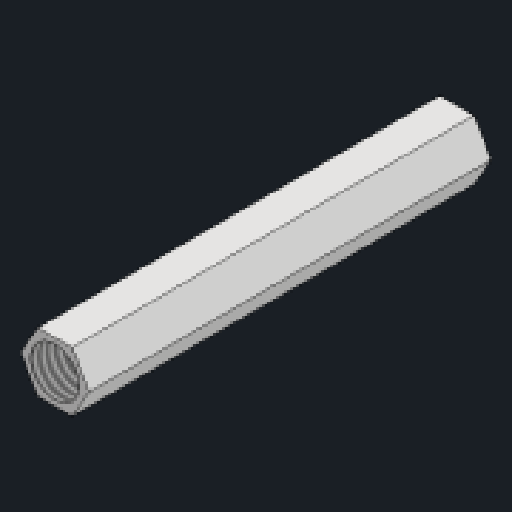
# Autodesk Inventor part: M3 x 25mm Threaded Spacer
Saved by Autodesk Inventor 2023.2 (Build 272271030, 271C)
## iProperties
Created: 2024-02-28
Part Number: M3 x 25mm Threaded Spacer
Material: Brass, Soft Yellow
Document SubType Name: Modeling
Designer: robpl
Density: 8.47 g/cm^3
Appearance: Brass - Satin
Author: robpl
Autodesk Inventor part; units mm, degrees
ref_plane "YZ Plane" through (0, 0, 0) normal (1, 0, 0) x (0, 1, 0)
ref_plane "XZ Plane" through (0, 0, 0) normal (0, 1, 0) x (-1, 0, 0)
ref_plane "XY Plane" through (0, 0, 0) normal (0, 0, 1) x (1, 0, 0)
sketch "Sketch1" plane through (0, 0, 0) normal (0, 0, 1) x (1, 0, 0)
  line L0 (-1.0681, -1.85) -> (-2.1362, 0)
  line L1 (-2.1362, 0) -> (-1.0681, 1.85)
  line L2 (-1.0681, 1.85) -> (1.0681, 1.85)
  line L3 (1.0681, 1.85) -> (2.1362, 0)
  line L4 (2.1362, 0) -> (1.0681, -1.85)
  line L5 (1.0681, -1.85) -> (-1.0681, -1.85)
  circle A0 centre (0, 0) radius 1.5
  dimension "d0" = 3.7
  dimension "d3" = 3
  constraints: 12 end point, 2 coincident, 1 centre point, 1 horizontal, 13 other
  measures "d0" distance between parallel lines of L2 L5
  measures "d3" diameter of A0
extrude "Extrusion1" add sketch "Sketch1" along normal mid plane 25
thread "Thread1" size "M3x0.5" class "6H" standard "ANSI Metric M Profile" full length
body "Solid1"
